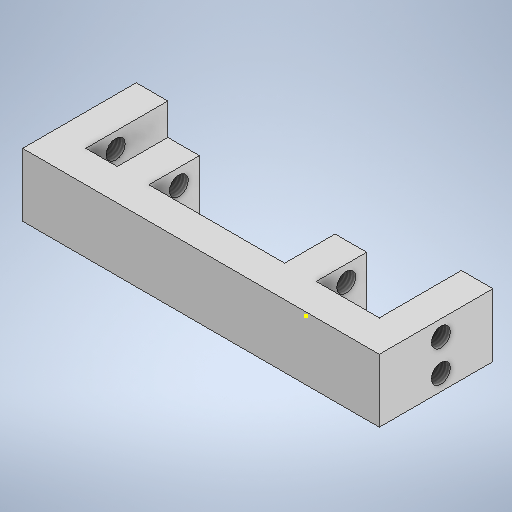
# Autodesk Inventor part: soporte
Saved by Autodesk Inventor 2025.2 (Build 292293000, 293)
## iProperties
Created: 2025-04-07
Part Number: soporte
Material: Generic
Document SubType Name: Modeling
Designer: maqmat
Density: 1 g/cm^3
Appearance: Default
Author: maqmat
Autodesk Inventor part; units mm, degrees
ref_plane "YZ Plane" through (0, 0, 0) normal (1, 0, 0) x (0, 1, 0)
ref_plane "XZ Plane" through (0, 0, 0) normal (0, 1, 0) x (-1, 0, 0)
ref_plane "XY Plane" through (0, 0, 0) normal (0, 0, 1) x (1, 0, 0)
sketch "Sketch1" plane through (0, 0, 0) normal (0, 1, 0) x (-1, 0, 0)
  line L0 (-6.122, -0.5654) -> (40.378, -0.5654)
  line L1 (40.378, -0.5654) -> (40.378, -5.5654)
  line L2 (40.378, -5.5654) -> (-6.122, -5.5654)
  line L3 (-6.122, -5.5654) -> (-6.122, -0.5654)
  line L4 (40.378, -0.5654) -> (45.378, -0.5654)
  line L5 (45.378, -0.5654) -> (45.378, -5.5654)
  line L6 (45.378, -5.5654) -> (40.378, -5.5654)
  line L7 (45.378, -5.5654) -> (45.378, -13.5654)
  line L8 (45.378, -13.5654) -> (40.378, -13.5654)
  line L9 (40.378, -13.5654) -> (40.378, -5.5654)
  line L10 (35.378, -13.5654) -> (35.378, -5.5654)
  line L11 (35.378, -13.5654) -> (30.378, -13.5654)
  line L12 (30.378, -13.5654) -> (30.378, -5.5654)
  line L13 (-6.122, -0.5654) -> (-11.122, -0.5654)
  line L14 (-11.122, -0.5654) -> (-11.122, -5.5654)
  line L15 (-11.122, -5.5654) -> (-6.122, -5.5654)
  line L16 (-11.122, -5.5654) -> (-11.122, -13.5654)
  line L17 (-11.122, -13.5654) -> (-6.122, -13.5654)
  line L18 (-6.122, -5.5654) -> (3.878, -5.5654)
  line L19 (3.878, -5.5654) -> (3.878, -13.5654)
  line L20 (3.878, -13.5654) -> (8.878, -13.5654)
  line L21 (8.878, -13.5654) -> (8.878, -5.5654)
  line L22 (-6.122, -5.5654) -> (-6.122, -13.5654)
  point P0 (0, 0)
  dimension "d0" = 46.5
  dimension "d1" = 5
  dimension "d2" = 5
  dimension "d3" = 8
  dimension "d4" = 5
  dimension "d5" = 5
  dimension "d6" = 5
  dimension "d7" = 8
  dimension "d8" = 10
  dimension "d9" = 5
  constraints: 46 end point, 14 perpendicular, 13 point on line, 2 horizontal, 1 vertical
  measures "d0" distance of L0.start L0.end
  measures "d1" distance of L0.end L1.end
  measures "d2" distance of L0.end L4.end
  measures "d3" distance of L5.end L7.end
  measures "d4" distance of L8.end L10.start
  measures "d5" distance of L10.start L11.end
  measures "d6" distance of L0.start L13.end
  measures "d7" distance of L14.end L16.end
  measures "d8" distance of L2.end L18.end
  measures "d9" distance of L19.end L20.end
extrude "Extrusion1" add sketch "Sketch1" along normal blind 10
sketch "Sketch2" plane through (-45.378, 0, -13.5654) normal (-1, 0, 0) x (0, 0, 1)
  line L0 (0, 10) -> (13, 10) projected
  line L1 (13, 10) -> (0, 10)
  line L2 (0, 10) -> (6.5, 10)
  line L3 (0, 0) -> (8, 0) projected
  line L4 (6.5, 0) -> (6.5, 10)
  line L5 (6.5, 5) -> (0, 5)
  line L6 (0, 5) -> (3.25, 5)
  line L7 (3.25, 0) -> (3.25, 5)
  line L8 (3.25, 10) -> (3.25, 5)
  circle A0 centre (3.25, 7.5) radius 1.5
  circle A1 centre (3.25, 2.5) radius 1.5
  point P0 (13.5654, 0)
  dimension "d12" = 3
  dimension "d13" = 3
  constraints: 14 end point, 6 midpoint, 2 centre point, 2 collinear, 2 perpendicular, 1 horizontal, 1 point on line
  measures "d12" diameter of A0
  measures "d13" diameter of A1
extrude "Extrusion2" cut sketch "Sketch2" against normal blind 60 contours A0 L8 | L8 A0 | A1 L7 | L7 A1
thread "Thread1" size "M3x0.5" class "6H" standard "ANSI Metric M Profile" full length
thread "Thread2" size "M3x0.5" class "6H" standard "ANSI Metric M Profile" full length
thread "Thread3" size "M3x0.5" class "6H" standard "ANSI Metric M Profile" full length
thread "Thread4" size "M3x0.5" class "6H" standard "ANSI Metric M Profile" full length
thread "Thread5" size "M3x0.5" class "6H" standard "ANSI Metric M Profile" full length
thread "Thread6" size "M3x0.5" class "6H" standard "ANSI Metric M Profile" full length
thread "Thread7" size "M3x0.5" class "6H" standard "ANSI Metric M Profile" full length
thread "Thread8" size "M3x0.5" class "6H" standard "ANSI Metric M Profile" full length
sketch "Sketch3" plane through (-40.378, 0, -13.5654) normal (0, 0, -1) x (-1, 0, 0)
  line L0 (5, 10) -> (-51.5, 10) projected
  line L1 (5, 0) -> (5, 10) projected
  line L2 (0.1606, 10) -> (5, 10)
  line L3 (5, 10) -> (5, 0)
  line L4 (5, 0) -> (0.1606, 0)
  line L5 (0.1606, 0) -> (0.1606, 10)
  line L6 (-10, 0) -> (-10, 10) projected
  line L7 (-5, 0) -> (-5, 10) projected
  line L8 (-10, 10) -> (-5, 10)
  line L9 (-5, 10) -> (-5, 0)
  line L10 (-5, 0) -> (-10, 0)
  line L11 (-10, 0) -> (-10, 10)
  line L12 (-36.5, 0) -> (-36.5, 10) projected
  line L13 (-31.5, 0) -> (-31.5, 10) projected
  line L14 (-36.5, 10) -> (-31.5, 10)
  line L15 (-31.5, 10) -> (-31.5, 0)
  line L16 (-31.5, 0) -> (-36.5, 0)
  line L17 (-36.5, 0) -> (-36.5, 10)
  line L18 (-46.5, 0) -> (-46.5, 10) projected
  line L19 (-51.5, 0) -> (-51.5, 10) projected
  line L20 (-46.5, 0) -> (-51.5, 0)
  line L21 (-51.5, 0) -> (-51.5, 10)
  line L22 (-51.5, 10) -> (-46.5, 10)
  line L23 (-46.5, 10) -> (-46.5, 0)
  line L24 (0, 10) -> (5, 10)
  line L25 (5, 10) -> (5, 0)
  line L26 (5, 0) -> (0, 0)
  line L27 (0, 0) -> (0, 10)
  point P0 (-40.378, 0)
  constraints: 40 end point, 10 parallel, 5 horizontal, 5 perpendicular, 2 other
extrude "Extrusion3" add sketch "Sketch3" along normal blind 5 contours L1 L4 L5 L0 | L18 L20 L19 L0 | L5 L26 L27 L0
sketch "Sketch4" plane through (0, 10, 0) normal (0, 1, 0) x (1, 0, 0)
  point P0 (0, 0)
body "Solid1"
